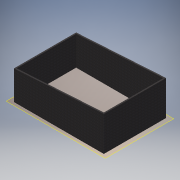
# Autodesk Inventor part: Wände
Saved by Autodesk Inventor 2017 (Build 210142000, 142)
## iProperties
Created: 2017-05-11
Part Number: Wände
Material: Beton
Document SubType Name: Modeling
Designer: Fake
Mass: 1.03996e+07 g
Surface Area: 907200 cm^2
Volume: 4.32e+06 cm^3
Density: 2.40731 g/cm^3
Appearance: Waschbeton - Grob
Author: Fake
Autodesk Inventor part; units mm, degrees
ref_plane "YZ Plane" through (0, 0, 0) normal (1, 0, 0) x (0, 1, 0)
ref_plane "XZ Plane" through (0, 0, 0) normal (0, 1, 0) x (-1, 0, 0)
ref_plane "XY Plane" through (0, 0, 0) normal (0, 0, 1) x (1, 0, 0)
ref_plane "Arbeitsebene1" through (0, 0, 0) normal (0, 0, 1) x (1, 0, 0)
sketch "Skizze1" plane through (0, 0, 0) normal (0, 0, 1) x (1, 0, 0)
  line L0 (-2500, 1500) -> (2500, 1500) projected
  line L1 (-2500, -1500) -> (-2500, 1500) projected
  line L2 (2500, -1500) -> (-2500, -1500) projected
  line L3 (2500, 1500) -> (2500, -1500) projected
  line L4 (-2400, 1400) -> (2400, 1400)
  line L5 (2400, 1400) -> (2400, -1400)
  line L6 (2400, -1400) -> (-2400, -1400)
  line L7 (-2400, -1400) -> (-2400, 1400)
  dimension "d0" = 100
  constraints: 8 end point, 3 other
  measures "d0" distance between parallel lines of L7 L1
extrude "Extrusion1" add sketch "Skizze1" along normal blind 2500
sketch "Skizze3" plane through (-2500, -1500, 0) normal (0, -1, 0) x (1, 0, 0)
  line L0 (5000, 0) -> (0, 0) projected
  line L1 (5000, 0) -> (5000, 2500) projected
  line L2 (0, 2500) -> (5000, 2500) projected
  line L3 (0, 0) -> (0, 2500) projected
  line L4 (5000, 0) -> (5000, 2500) projected
  line L5 (5000, 2500) -> (0, 2100)
  line L6 (0, 0) -> (0, 2500) projected
  line L7 (0, 2500) -> (0, 2100)
  line L8 (0, 2500) -> (5000, 2500) projected
  line L9 (0, 2500) -> (5000, 2500)
  dimension "d11" = 400
  constraints: 6 end point, 2 collinear, 1 point on line
  measures "d11" distance of L2.start L5.end
extrude "Extrusion3" cut sketch "Skizze3" against normal up to surface (3000 mm away) contours L5 L3 L2
sketch "Skizze2" plane through (-2500, -1500, 0) normal (0, -1, 0) x (1, 0, 0)
  line L0 (5000, 0) -> (0, 0) projected
  line L1 (5000, 0) -> (5000, 2500) projected
  line L2 (0, 0) -> (0, 2100) projected
  line L3 (1000, 0) -> (2200, 0)
  line L4 (2200, 0) -> (2200, 1800)
  line L5 (2200, 1800) -> (1000, 1800)
  line L6 (1000, 1800) -> (1000, 0)
  line L7 (0, 0) -> (5000, 0) projected
  line L8 (3000, 0) -> (4500, 0)
  line L9 (4500, 0) -> (4500, 1800)
  line L10 (4500, 1800) -> (3000, 1800)
  line L11 (3000, 1800) -> (3000, 0)
  line L12 (5000, 2500) -> (0, 2100) projected
  dimension "d3" = 1800
  dimension "d4" = 1500
  dimension "d5" = 1200
  dimension "d6" = 500
  dimension "d7" = 1000
  constraints: 16 end point, 4 parallel, 3 point on line, 2 horizontal, 2 perpendicular
  measures "d3" distance between parallel lines of L0 L10
  measures "d4" distance of L9.end L10.end
  measures "d5" distance of L4.end L5.end
  measures "d6" distance between parallel lines of L1 L9
  measures "d7" distance between parallel lines of L2 L6
extrude "Extrusion2" cut sketch "Skizze2" against normal blind 396.5 contours L0 L11 L10 L9 | L0 L6 L5 L4
